Autodesk Inventor part; units mm, degrees
(part 2 of 4)
  line L908 (-4.5, 107.4545) -> (-3, 104.8564)
  line L909 (-7.5, 107.4545) -> (-4.5, 107.4545)
  line L910 (-9, 104.8564) -> (-7.5, 107.4545)
  line L911 (-11.5, 100.5263) -> (-8.5, 100.5263)
  line L912 (-3, 91) -> (-3, 104.8564) construction
  line L913 (-80.5, 109.3301) -> (-83.5, 109.3301)
  line L914 (-83.5, 109.3301) -> (-85, 111.9282)
  line L915 (-85, 111.9282) -> (-83.5, 114.5263)
  line L916 (-83.5, 114.5263) -> (-80.5, 114.5263)
  line L917 (-72.5, 109.3301) -> (-75.5, 109.3301)
  line L918 (-75.5, 109.3301) -> (-77, 111.9282)
  line L919 (-80.5, 114.5263) -> (-79, 111.9282)
  line L920 (-77, 111.9282) -> (-75.5, 114.5263)
  line L921 (-71, 111.9282) -> (-72.5, 109.3301)
  line L922 (-75.5, 114.5263) -> (-72.5, 114.5263)
  line L923 (-72.5, 114.5263) -> (-71, 111.9282)
  line L924 (-79, 111.9282) -> (-80.5, 109.3301)
  line L925 (-51.5, 114.5263) -> (-48.5, 114.5263)
  line L926 (-48.5, 109.3301) -> (-51.5, 109.3301)
  line L927 (-51.5, 109.3301) -> (-53, 111.9282)
  line L928 (-53, 111.9282) -> (-51.5, 114.5263)
  line L929 (-56.5, 114.5263) -> (-55, 111.9282)
  line L930 (-55, 111.9282) -> (-56.5, 109.3301)
  line L931 (-56.5, 109.3301) -> (-59.5, 109.3301)
  line L932 (-59.5, 114.5263) -> (-56.5, 114.5263)
  line L933 (-61, 111.9282) -> (-59.5, 114.5263)
  line L934 (-64.5, 114.5263) -> (-63, 111.9282)
  line L935 (-63, 111.9282) -> (-64.5, 109.3301)
  line L936 (-67.5, 114.5263) -> (-64.5, 114.5263)
  line L937 (-64.5, 109.3301) -> (-67.5, 109.3301)
  line L938 (-69, 111.9282) -> (-67.5, 114.5263)
  line L939 (-67.5, 109.3301) -> (-69, 111.9282)
  line L940 (-59.5, 109.3301) -> (-61, 111.9282)
  line L941 (-76.5, 116.2583) -> (-79.5, 116.2583)
  line L942 (-79.5, 116.2583) -> (-81, 118.8564)
  line L943 (-79.5, 121.4545) -> (-76.5, 121.4545)
  line L944 (-81, 118.8564) -> (-79.5, 121.4545)
  line L945 (-39.5, 116.2583) -> (-41, 118.8564)
  line L946 (-41, 118.8564) -> (-39.5, 121.4545)
  line L947 (-43, 118.8564) -> (-44.5, 116.2583)
  line L948 (-44.5, 121.4545) -> (-43, 118.8564)
  line L949 (-47.5, 121.4545) -> (-44.5, 121.4545)
  line L950 (-49, 118.8564) -> (-47.5, 121.4545)
  line L951 (-47.5, 116.2583) -> (-49, 118.8564)
  line L952 (-52.5, 121.4545) -> (-51, 118.8564)
  line L953 (-51, 118.8564) -> (-52.5, 116.2583)
  line L954 (-55.5, 121.4545) -> (-52.5, 121.4545)
  line L955 (-52.5, 116.2583) -> (-55.5, 116.2583)
  line L956 (-44.5, 116.2583) -> (-47.5, 116.2583)
  line L957 (-57, 118.8564) -> (-55.5, 121.4545)
  line L958 (-60.5, 121.4545) -> (-59, 118.8564)
  line L959 (-59, 118.8564) -> (-60.5, 116.2583)
  line L960 (-63.5, 121.4545) -> (-60.5, 121.4545)
  line L961 (-60.5, 116.2583) -> (-63.5, 116.2583)
  line L962 (-63.5, 116.2583) -> (-65, 118.8564)
  line L963 (-65, 118.8564) -> (-63.5, 121.4545)
  line L964 (-55.5, 116.2583) -> (-57, 118.8564)
  line L965 (-67, 118.8564) -> (-68.5, 116.2583)
  line L966 (-68.5, 121.4545) -> (-67, 118.8564)
  line L967 (-68.5, 116.2583) -> (-71.5, 116.2583)
  line L968 (-71.5, 116.2583) -> (-73, 118.8564)
  line L969 (-73, 118.8564) -> (-71.5, 121.4545)
  line L970 (-75, 118.8564) -> (-76.5, 116.2583)
  line L971 (-76.5, 121.4545) -> (-75, 118.8564)
  line L972 (-71.5, 121.4545) -> (-68.5, 121.4545)
  line L973 (-47, 111.9282) -> (-48.5, 109.3301)
  line L974 (-48.5, 114.5263) -> (-47, 111.9282)
  line L975 (-45, 111.9282) -> (-43.5, 114.5263)
  line L976 (-43.5, 109.3301) -> (-45, 111.9282)
  line L977 (-43.5, 114.5263) -> (-40.5, 114.5263)
  line L978 (-40.5, 109.3301) -> (-43.5, 109.3301)
  line L979 (-40.5, 114.5263) -> (-39, 111.9282)
  line L980 (-39, 111.9282) -> (-40.5, 109.3301)
  line L981 (-11, 118.8564) -> (-12.5, 116.2583)
  line L982 (-12.5, 121.4545) -> (-11, 118.8564)
  line L983 (-24.5, 114.5263) -> (-23, 111.9282)
  line L984 (-23, 111.9282) -> (-24.5, 109.3301)
  line L985 (-27.5, 114.5263) -> (-24.5, 114.5263)
  line L986 (-24.5, 109.3301) -> (-27.5, 109.3301)
  line L987 (-29, 111.9282) -> (-27.5, 114.5263)
  line L988 (-27.5, 109.3301) -> (-29, 111.9282)
  line L989 (-31, 111.9282) -> (-32.5, 109.3301)
  line L990 (-32.5, 114.5263) -> (-31, 111.9282)
  line L991 (-32.5, 109.3301) -> (-35.5, 109.3301)
  line L992 (-35.5, 114.5263) -> (-32.5, 114.5263)
  line L993 (-35.5, 109.3301) -> (-37, 111.9282)
  line L994 (-37, 111.9282) -> (-35.5, 114.5263)
  line L995 (-19.5, 109.3301) -> (-21, 111.9282)
  line L996 (-21, 111.9282) -> (-19.5, 114.5263)
  line L997 (-19.5, 114.5263) -> (-16.5, 114.5263)
  line L998 (-16.5, 109.3301) -> (-19.5, 109.3301)
  line L999 (-16.5, 114.5263) -> (-15, 111.9282)
  line L1000 (-15, 111.9282) -> (-16.5, 109.3301)
  line L1001 (-20.5, 116.2583) -> (-23.5, 116.2583)
  line L1002 (-23.5, 121.4545) -> (-20.5, 121.4545)
  line L1003 (-19, 118.8564) -> (-20.5, 116.2583)
  line L1004 (-20.5, 121.4545) -> (-19, 118.8564)
  line L1005 (-17, 118.8564) -> (-15.5, 121.4545)
  line L1006 (-15.5, 116.2583) -> (-17, 118.8564)
  line L1007 (-12.5, 116.2583) -> (-15.5, 116.2583)
  line L1008 (-15.5, 121.4545) -> (-12.5, 121.4545)
  line L1009 (-25, 118.8564) -> (-23.5, 121.4545)
  line L1010 (-28.5, 121.4545) -> (-27, 118.8564)
  line L1011 (-27, 118.8564) -> (-28.5, 116.2583)
  line L1012 (-31.5, 121.4545) -> (-28.5, 121.4545)
  line L1013 (-28.5, 116.2583) -> (-31.5, 116.2583)
  line L1014 (-33, 118.8564) -> (-31.5, 121.4545)
  line L1015 (-31.5, 116.2583) -> (-33, 118.8564)
  line L1016 (-23.5, 116.2583) -> (-25, 118.8564)
  line L1017 (-36.5, 121.4545) -> (-35, 118.8564)
  line L1018 (-35, 118.8564) -> (-36.5, 116.2583)
  line L1019 (-39.5, 121.4545) -> (-36.5, 121.4545)
  line L1020 (-36.5, 116.2583) -> (-39.5, 116.2583)
  line L1021 (-13, 111.9282) -> (-11.5, 114.5263)
  line L1022 (-8.5, 109.3301) -> (-11.5, 109.3301)
  line L1023 (-11.5, 109.3301) -> (-13, 111.9282)
  line L1024 (-8.5, 114.5263) -> (-7, 111.9282)
  line L1025 (-7, 111.9282) -> (-8.5, 109.3301)
  line L1026 (-4.5, 116.2583) -> (-7.5, 116.2583)
  line L1027 (-7.5, 116.2583) -> (-9, 118.8564)
  line L1028 (-3, 118.8564) -> (-4.5, 116.2583)
  line L1029 (-4.5, 121.4545) -> (-3, 118.8564)
  line L1030 (-7.5, 121.4545) -> (-4.5, 121.4545)
  line L1031 (-9, 118.8564) -> (-7.5, 121.4545)
  line L1032 (-11.5, 114.5263) -> (-8.5, 114.5263)
  line L1033 (-3, 105) -> (-3, 118.8564) construction
  line L1034 (-80.5, 123.3301) -> (-83.5, 123.3301)
  line L1035 (-83.5, 123.3301) -> (-85, 125.9282)
  line L1036 (-85, 125.9282) -> (-83.5, 128.5263)
  line L1037 (-83.5, 128.5263) -> (-80.5, 128.5263)
  line L1038 (-72.5, 123.3301) -> (-75.5, 123.3301)
  line L1039 (-75.5, 123.3301) -> (-77, 125.9282)
  line L1040 (-80.5, 128.5263) -> (-79, 125.9282)
  line L1041 (-77, 125.9282) -> (-75.5, 128.5263)
  line L1042 (-71, 125.9282) -> (-72.5, 123.3301)
  line L1043 (-75.5, 128.5263) -> (-72.5, 128.5263)
  line L1044 (-72.5, 128.5263) -> (-71, 125.9282)
  line L1045 (-79, 125.9282) -> (-80.5, 123.3301)
  line L1046 (-51.5, 128.5263) -> (-48.5, 128.5263)
  line L1047 (-48.5, 123.3301) -> (-51.5, 123.3301)
  line L1048 (-51.5, 123.3301) -> (-53, 125.9282)
  line L1049 (-53, 125.9282) -> (-51.5, 128.5263)
  line L1050 (-56.5, 128.5263) -> (-55, 125.9282)
  line L1051 (-55, 125.9282) -> (-56.5, 123.3301)
  line L1052 (-56.5, 123.3301) -> (-59.5, 123.3301)
  line L1053 (-59.5, 128.5263) -> (-56.5, 128.5263)
  line L1054 (-61, 125.9282) -> (-59.5, 128.5263)
  line L1055 (-64.5, 128.5263) -> (-63, 125.9282)
  line L1056 (-63, 125.9282) -> (-64.5, 123.3301)
  line L1057 (-67.5, 128.5263) -> (-64.5, 128.5263)
  line L1058 (-64.5, 123.3301) -> (-67.5, 123.3301)
  line L1059 (-69, 125.9282) -> (-67.5, 128.5263)
  line L1060 (-67.5, 123.3301) -> (-69, 125.9282)
  line L1061 (-59.5, 123.3301) -> (-61, 125.9282)
  line L1062 (-76.5, 130.2583) -> (-79.5, 130.2583)
  line L1063 (-79.5, 130.2583) -> (-81, 132.8564)
  line L1064 (-79.5, 135.4545) -> (-76.5, 135.4545)
  line L1065 (-81, 132.8564) -> (-79.5, 135.4545)
  line L1066 (-39.5, 130.2583) -> (-41, 132.8564)
  line L1067 (-41, 132.8564) -> (-39.5, 135.4545)
  line L1068 (-43, 132.8564) -> (-44.5, 130.2583)
  line L1069 (-44.5, 135.4545) -> (-43, 132.8564)
  line L1070 (-47.5, 135.4545) -> (-44.5, 135.4545)
  line L1071 (-49, 132.8564) -> (-47.5, 135.4545)
  line L1072 (-47.5, 130.2583) -> (-49, 132.8564)
  line L1073 (-52.5, 135.4545) -> (-51, 132.8564)
  line L1074 (-51, 132.8564) -> (-52.5, 130.2583)
  line L1075 (-55.5, 135.4545) -> (-52.5, 135.4545)
  line L1076 (-52.5, 130.2583) -> (-55.5, 130.2583)
  line L1077 (-44.5, 130.2583) -> (-47.5, 130.2583)
  line L1078 (-57, 132.8564) -> (-55.5, 135.4545)
  line L1079 (-60.5, 135.4545) -> (-59, 132.8564)
  line L1080 (-59, 132.8564) -> (-60.5, 130.2583)
  line L1081 (-63.5, 135.4545) -> (-60.5, 135.4545)
  line L1082 (-60.5, 130.2583) -> (-63.5, 130.2583)
  line L1083 (-63.5, 130.2583) -> (-65, 132.8564)
  line L1084 (-65, 132.8564) -> (-63.5, 135.4545)
  line L1085 (-55.5, 130.2583) -> (-57, 132.8564)
  line L1086 (-67, 132.8564) -> (-68.5, 130.2583)
  line L1087 (-68.5, 135.4545) -> (-67, 132.8564)
  line L1088 (-68.5, 130.2583) -> (-71.5, 130.2583)
  line L1089 (-71.5, 130.2583) -> (-73, 132.8564)
  line L1090 (-73, 132.8564) -> (-71.5, 135.4545)
  line L1091 (-75, 132.8564) -> (-76.5, 130.2583)
  line L1092 (-76.5, 135.4545) -> (-75, 132.8564)
  line L1093 (-71.5, 135.4545) -> (-68.5, 135.4545)
  line L1094 (-47, 125.9282) -> (-48.5, 123.3301)
  line L1095 (-48.5, 128.5263) -> (-47, 125.9282)
  line L1096 (-45, 125.9282) -> (-43.5, 128.5263)
  line L1097 (-43.5, 123.3301) -> (-45, 125.9282)
  line L1098 (-43.5, 128.5263) -> (-40.5, 128.5263)
  line L1099 (-40.5, 123.3301) -> (-43.5, 123.3301)
  line L1100 (-40.5, 128.5263) -> (-39, 125.9282)
  line L1101 (-39, 125.9282) -> (-40.5, 123.3301)
  line L1102 (-11, 132.8564) -> (-12.5, 130.2583)
  line L1103 (-12.5, 135.4545) -> (-11, 132.8564)
  line L1104 (-24.5, 128.5263) -> (-23, 125.9282)
  line L1105 (-23, 125.9282) -> (-24.5, 123.3301)
  line L1106 (-27.5, 128.5263) -> (-24.5, 128.5263)
  line L1107 (-24.5, 123.3301) -> (-27.5, 123.3301)
  line L1108 (-29, 125.9282) -> (-27.5, 128.5263)
  line L1109 (-27.5, 123.3301) -> (-29, 125.9282)
  line L1110 (-31, 125.9282) -> (-32.5, 123.3301)
  line L1111 (-32.5, 128.5263) -> (-31, 125.9282)
  line L1112 (-32.5, 123.3301) -> (-35.5, 123.3301)
  line L1113 (-35.5, 128.5263) -> (-32.5, 128.5263)
  line L1114 (-35.5, 123.3301) -> (-37, 125.9282)
  line L1115 (-37, 125.9282) -> (-35.5, 128.5263)
  line L1116 (-19.5, 123.3301) -> (-21, 125.9282)
  line L1117 (-21, 125.9282) -> (-19.5, 128.5263)
  line L1118 (-19.5, 128.5263) -> (-16.5, 128.5263)
  line L1119 (-16.5, 123.3301) -> (-19.5, 123.3301)
  line L1120 (-16.5, 128.5263) -> (-15, 125.9282)
  line L1121 (-15, 125.9282) -> (-16.5, 123.3301)
  line L1122 (-20.5, 130.2583) -> (-23.5, 130.2583)
  line L1123 (-23.5, 135.4545) -> (-20.5, 135.4545)
  line L1124 (-19, 132.8564) -> (-20.5, 130.2583)
  line L1125 (-20.5, 135.4545) -> (-19, 132.8564)
  line L1126 (-17, 132.8564) -> (-15.5, 135.4545)
  line L1127 (-15.5, 130.2583) -> (-17, 132.8564)
  line L1128 (-12.5, 130.2583) -> (-15.5, 130.2583)
  line L1129 (-15.5, 135.4545) -> (-12.5, 135.4545)
  line L1130 (-25, 132.8564) -> (-23.5, 135.4545)
  line L1131 (-28.5, 135.4545) -> (-27, 132.8564)
  line L1132 (-27, 132.8564) -> (-28.5, 130.2583)
  line L1133 (-31.5, 135.4545) -> (-28.5, 135.4545)
  line L1134 (-28.5, 130.2583) -> (-31.5, 130.2583)
  line L1135 (-33, 132.8564) -> (-31.5, 135.4545)
  line L1136 (-31.5, 130.2583) -> (-33, 132.8564)
  line L1137 (-23.5, 130.2583) -> (-25, 132.8564)
  line L1138 (-36.5, 135.4545) -> (-35, 132.8564)
  line L1139 (-35, 132.8564) -> (-36.5, 130.2583)
  line L1140 (-39.5, 135.4545) -> (-36.5, 135.4545)
  line L1141 (-36.5, 130.2583) -> (-39.5, 130.2583)
  line L1142 (-13, 125.9282) -> (-11.5, 128.5263)
  line L1143 (-8.5, 123.3301) -> (-11.5, 123.3301)
  line L1144 (-11.5, 123.3301) -> (-13, 125.9282)
  line L1145 (-8.5, 128.5263) -> (-7, 125.9282)
  line L1146 (-7, 125.9282) -> (-8.5, 123.3301)
  line L1147 (-4.5, 130.2583) -> (-7.5, 130.2583)
  line L1148 (-7.5, 130.2583) -> (-9, 132.8564)
  line L1149 (-3, 132.8564) -> (-4.5, 130.2583)
  line L1150 (-4.5, 135.4545) -> (-3, 132.8564)
  line L1151 (-7.5, 135.4545) -> (-4.5, 135.4545)
  line L1152 (-9, 132.8564) -> (-7.5, 135.4545)
  line L1153 (-11.5, 128.5263) -> (-8.5, 128.5263)
  line L1154 (-3, 119) -> (-3, 132.8564) construction
  point P0 (0, 75)
  point P1 (-6, 7)
  point P2 (-14, 7)
  point P3 (-22, 7)
  point P4 (-30, 7)
  point P5 (-38, 7)
  point P6 (-46, 7)
  point P7 (-54, 7)
  point P8 (-62, 7)
  point P9 (-70, 7)
  point P10 (-78, 7)
  point P11 (-10, 13.9282)
  point P12 (-18, 13.9282)
  point P13 (-26, 13.9282)
  point P14 (-34, 13.9282)
  point P15 (-42, 13.9282)
  point P16 (-50, 13.9282)
  point P17 (-58, 13.9282)
  point P18 (-66, 13.9282)
  point P19 (-74, 13.9282)
  point P20 (-82, 13.9282)
  point P21 (-14, 20.8564)
  point P22 (-22, 20.8564)
  point P23 (-30, 20.8564)
  point P24 (-38, 20.8564)
  point P25 (-46, 20.8564)
  point P26 (-54, 20.8564)
  point P27 (-62, 20.8564)
  point P28 (-70, 20.8564)
  point P29 (-78, 20.8564)
  point P30 (-86, 20.8564)
  point P31 (-6, 20.8564)
  point P32 (-82, 27.9282)
  point P33 (-74, 27.9282)
  point P34 (-50, 27.9282)
  point P35 (-58, 27.9282)
  point P36 (-66, 27.9282)
  point P37 (-84.5, 32.2583)
  point P38 (-83, 34.8564)
  point P39 (-86, 34.8564)
  point P40 (-84.5, 37.4545)
  point P41 (-78, 34.8564)
  point P42 (-46, 34.8564)
  point P43 (-54, 34.8564)
  point P44 (-62, 34.8564)
  point P45 (-70, 34.8564)
  point P46 (-42, 27.9282)
  point P47 (-26, 27.9282)
  point P48 (-34, 27.9282)
  point P49 (-18, 27.9282)
  point P50 (-14, 34.8564)
  point P51 (-22, 34.8564)
  point P52 (-30, 34.8564)
  point P53 (-38, 34.8564)
  point P54 (-10, 27.9282)
  point P55 (-6, 34.8564)
  point P56 (-82, 41.9282)
  point P57 (-74, 41.9282)
  point P58 (-50, 41.9282)
  point P59 (-58, 41.9282)
  point P60 (-66, 41.9282)
  point P61 (-84.5, 46.2583)
  point P62 (-83, 48.8564)
  point P63 (-86, 48.8564)
  point P64 (-84.5, 51.4545)
  point P65 (-78, 48.8564)
  point P66 (-46, 48.8564)
  point P67 (-54, 48.8564)
  point P68 (-62, 48.8564)
  point P69 (-70, 48.8564)
  point P70 (-42, 41.9282)
  point P71 (-26, 41.9282)
  point P72 (-34, 41.9282)
  point P73 (-18, 41.9282)
  point P74 (-14, 48.8564)
  point P75 (-22, 48.8564)
  point P76 (-30, 48.8564)
  point P77 (-38, 48.8564)
  point P78 (-10, 41.9282)
  point P79 (-6, 48.8564)
  point P80 (-82, 55.9282)
  point P81 (-74, 55.9282)
  point P82 (-50, 55.9282)
  point P83 (-58, 55.9282)
  point P84 (-66, 55.9282)
  point P85 (-84.5, 60.2583)
  point P86 (-83, 62.8564)
  point P87 (-86, 62.8564)
  point P88 (-84.5, 65.4545)
  point P89 (-78, 62.8564)
  point P90 (-46, 62.8564)
  point P91 (-54, 62.8564)
  point P92 (-62, 62.8564)
  point P93 (-70, 62.8564)
  point P94 (-42, 55.9282)
  point P95 (-26, 55.9282)
  point P96 (-34, 55.9282)
  point P97 (-18, 55.9282)
  point P98 (-14, 62.8564)
  point P99 (-22, 62.8564)
  point P100 (-30, 62.8564)
  point P101 (-38, 62.8564)
  point P102 (-10, 55.9282)
  point P103 (-6, 62.8564)
  point P104 (-82, 69.9282)
  point P105 (-74, 69.9282)
  point P106 (-50, 69.9282)
  point P107 (-58, 69.9282)
  point P108 (-66, 69.9282)
  point P109 (-84.5, 74.2583)
  point P110 (-83, 76.8564)
  point P111 (-86, 76.8564)
  point P112 (-84.5, 79.4545)
  point P113 (-78, 76.8564)
  point P114 (-46, 76.8564)
  point P115 (-54, 76.8564)
  point P116 (-62, 76.8564)
  point P117 (-70, 76.8564)
  point P118 (-42, 69.9282)
  point P119 (-26, 69.9282)
  point P120 (-34, 69.9282)
  point P121 (-18, 69.9282)
  point P122 (-14, 76.8564)
  point P123 (-22, 76.8564)
  point P124 (-30, 76.8564)
  point P125 (-38, 76.8564)
  point P126 (-10, 69.9282)
  point P127 (-6, 76.8564)
  point P128 (-82, 83.9282)
  point P129 (-74, 83.9282)
  point P130 (-50, 83.9282)
  point P131 (-58, 83.9282)
  point P132 (-66, 83.9282)
  point P133 (-84.5, 88.2583)
  point P134 (-83, 90.8564)
  point P135 (-86, 90.8564)
  point P136 (-84.5, 93.4545)
  point P137 (-78, 90.8564)
  point P138 (-46, 90.8564)
  point P139 (-54, 90.8564)
  point P140 (-62, 90.8564)
  point P141 (-70, 90.8564)
  point P142 (-42, 83.9282)
  point P143 (-26, 83.9282)
  point P144 (-34, 83.9282)
  point P145 (-18, 83.9282)
  point P146 (-14, 90.8564)
  point P147 (-22, 90.8564)
  point P148 (-30, 90.8564)
  point P149 (-38, 90.8564)
  point P150 (-10, 83.9282)
  point P151 (-6, 90.8564)
  point P152 (-82, 97.9282)
  point P153 (-74, 97.9282)
  point P154 (-50, 97.9282)
  point P155 (-58, 97.9282)
  point P156 (-66, 97.9282)
  point P157 (-84.5, 102.2583)
  point P158 (-83, 104.8564)
  point P159 (-86, 104.8564)
  point P160 (-84.5, 107.4545)
  point P161 (-78, 104.8564)
  point P162 (-46, 104.8564)
  point P163 (-54, 104.8564)
  point P164 (-62, 104.8564)
  point P165 (-70, 104.8564)
  point P166 (-42, 97.9282)
  point P167 (-26, 97.9282)
  point P168 (-34, 97.9282)
  point P169 (-18, 97.9282)
  point P170 (-14, 104.8564)
  point P171 (-22, 104.8564)
  point P172 (-30, 104.8564)
  point P173 (-38, 104.8564)
  point P174 (-10, 97.9282)
  point P175 (-6, 104.8564)
  point P176 (-82, 111.9282)
  point P177 (-74, 111.9282)
  point P178 (-50, 111.9282)
  point P179 (-58, 111.9282)
  point P180 (-66, 111.9282)
  point P181 (-84.5, 116.2583)
  point P182 (-83, 118.8564)
  point P183 (-86, 118.8564)
  point P184 (-84.5, 121.4545)
  point P185 (-78, 118.8564)
  point P186 (-46, 118.8564)
  point P187 (-54, 118.8564)
  point P188 (-62, 118.8564)
  point P189 (-70, 118.8564)
  point P190 (-42, 111.9282)
  point P191 (-26, 111.9282)
  point P192 (-34, 111.9282)
  point P193 (-18, 111.9282)
  point P194 (-14, 118.8564)
  point P195 (-22, 118.8564)
  point P196 (-30, 118.8564)
  point P197 (-38, 118.8564)
  point P198 (-10, 111.9282)
  point P199 (-6, 118.8564)
  dimension "d22" = 3
  dimension "d25" = 8
  dimension "d28" = 8
  dimension "d33" = 8
  dimension "d40" = 14
  constraints: 2310 end point, 4 collinear, 2 horizontal, 2 vertical, 2528 other
  measures "d22" distance of point (-6, 7) L0.start
  measures "d25" distance of point (-6, 7) point (-14, 7)
  measures "d28" distance of point (-6, 7) point (-10, 13.928)
  measures "d33" distance of point (-14, 20.856) point (-6, 20.856)
  measures "d40" distance of L117.end L187.start
extrude "Estrusione3" cut sketch "Schizzo4" against normal blind 5 contours L12 L13 L14 L15 L16 L17 | L18 L19 L20 L21 L22 L23 | L24 L25 L26 L27 L28 L29 | L30 L31 L32 L33 L34 L35 | L36 L37 L38 L39 L40 L41 | L42 L43 L44 L45 L46 L47 | L48 L49 L50 L51 L52 L53 | L60 L61 L62 L63 L64 L65 | L66 L67 L68 L69 L70 L71 | L72 L73 L74 L75 L76 L77 | L78 L79 L80 L81 L82 L83 | L84 L85 L86 L87 L88 L89 | L90 L91 L92 L93 L94 L95 | L96 L97 L98 L99 L100 L101 | L102 L103 L104 L105 L106 L107 | L108 L109 L110 L111 L112 L113 | L114 L115 L116 L117 L118 L119 | L120 L121 L122 L123 L124 L125 | L126 L127 L128 L129 L130 L131 | L132 L133 L134 L135 L136 L137 | L138 L139 L140 L141 L142 L143 | L144 L145 L146 L147 L148 L149 | L150 L151 L152 L153 L154 L155 | L156 L157 L158 L159 L160 L161 | L162 L163 L164 L165 L166 L167 | L168 L169 L170 L171 L172 L173 | L180 L182 L185 L184 L183 L181 | L187 L188 L189 L190 L193 L198 | L191 L192 L194 L196 L197 L195 | L199 L248 L247 L200 L201 L202 | L203 L204 L205 L214 L207 L206 | L208 L209 L211 L213 L212 L210 | L215 L216 L218 L217 L245 L244 | L219 L220 L293 L291 L292 L294 | L221 L230 L225 L224 L223 L222 | L226 L227 L229 L238 L231 L228 | L232 L233 L235 L236 L237 L234 | L239 L241 L242 L243 L246 L240 | L249 L251 L253 L254 L252 L250 | L255 L281 L280 L279 L282 L256 | L257 L258 L260 L262 L261 L259 | L263 L265 L267 L268 L266 L264 | L269 L270 L271 L273 L274 L272 | L275 L290 L283 L276 L278 L277 | L284 L285 L287 L289 L288 L286 | L295 L306 L298 L299 L296 L297 | L300 L301 L305 L304 L303 L302 | L308 L309 L310 L311 L314 L319 | L312 L313 L315 L317 L318 L316 | L320 L369 L368 L321 L322 L323 | L324 L325 L326 L335 L328 L327 | L329 L330 L332 L334 L333 L331 | L336 L337 L339 L338 L366 L365 | L340 L341 L414 L412 L413 L415 | L342 L351 L346 L345 L344 L343 | L347 L348 L350 L359 L352 L349 | L353 L354 L356 L357 L358 L355 | L360 L362 L363 L364 L367 L361 | L370 L372 L374 L375 L373 L371 | L376 L402 L401 L400 L403 L377 | L378 L379 L381 L383 L382 L380 | L384 L386 L388 L389 L387 L385 | L390 L391 L392 L394 L395 L393 | L396 L411 L404 L397 L399 L398 | L405 L406 L408 L410 L409 L407 | L416 L427 L419 L420 L417 L418 | L421 L422 L426 L425 L424 L423 | L429 L430 L431 L432 L435 L440 | L433 L434 L436 L438 L439 L437 | L441 L490 L489 L442 L443 L444 | L445 L446 L447 L456 L449 L448 | L450 L451 L453 L455 L454 L452 | L457 L458 L460 L459 L487 L486 | L461 L462 L535 L533 L534 L536 | L463 L472 L467 L466 L465 L464 | L468 L469 L471 L480 L473 L470 | L474 L475 L477 L478 L479 L476 | L481 L483 L484 L485 L488 L482 | L491 L493 L495 L496 L494 L492 | L497 L523 L522 L521 L524 L498 | L499 L500 L502 L504 L503 L501 | L505 L507 L509 L510 L508 L506 | L511 L512 L513 L515 L516 L514 | L517 L532 L525 L518 L520 L519 | L526 L527 L529 L531 L530 L528 | L537 L548 L540 L541 L538 L539 | L542 L543 L547 L546 L545 L544 | L550 L551 L552 L553 L556 L561 | L554 L555 L557 L559 L560 L558 | L562 L611 L610 L563 L564 L565 | L566 L567 L568 L577 L570 L569 | L571 L572 L574 L576 L575 L573 | L578 L579 L581 L580 L608 L607 | L582 L583 L656 L654 L655 L657 | L584 L593 L588 L587 L586 L585 | L589 L590 L592 L601 L594 L591 | L595 L596 L598 L599 L600 L597 | L602 L604 L605 L606 L609 L603 | L612 L614 L616 L617 L615 L613 | L618 L644 L643 L642 L645 L619 | L620 L621 L623 L625 L624 L622 | L626 L628 L630 L631 L629 L627 | L632 L633 L634 L636 L637 L635 | L638 L653 L646 L639 L641 L640 | L647 L648 L650 L652 L651 L649 | L658 L669 L661 L662 L659 L660 | L663 L664 L668 L667 L666 L665 | L671 L672 L673 L674 L677 L682 | L675 L676 L678 L680 L681 L679 | L683 L732 L731 L684 L685 L686 | L687 L688 L689 L698 L691 L690 | L692 L693 L695 L697 L696 L694 | L699 L700 L702 L701 L729 L728 | L703 L704 L777 L775 L776 L778 | L705 L714 L709 L708 L707 L706 | L710 L711 L713 L722 L715 L712 | L716 L717 L719 L720 L721 L718 | L723 L725 L726 L727 L730 L724 | L733 L735 L737 L738 L736 L734 | L741 L742 L744 L746 L745 L743 | L747 L749 L751 L752 L750 L748 | L753 L754 L755 L757 L758 L756 | L779 L790 L782 L783 L780 L781 | L792 L793 L794 L795 L798 L803 | L796 L797 L799 L801 L802 L800 | L804 L853 L852 L805 L806 L807 | L808 L809 L810 L819 L812 L811 | L813 L814 L816 L818 L817 L815 | L820 L821 L823 L822 L850 L849 | L824 L825 L898 L896 L897 L899 | L826 L835 L830 L829 L828 L827 | L831 L832 L834 L843 L836 L833 | L837 L838 L840 L841 L842 L839 | L844 L846 L847 L848 L851 L845 | L854 L856 L858 L859 L857 L855 | L868 L870 L872 L873 L871 L869 | L913 L914 L915 L916 L919 L924 | L917 L918 L920 L922 L923 L921 | L925 L974 L973 L926 L927 L928 | L929 L930 L931 L940 L933 L932 | L934 L935 L937 L939 L938 L936 | L941 L942 L944 L943 L971 L970 | L945 L946 L1019 L1017 L1018 L1020 | L947 L956 L951 L950 L949 L948 | L952 L953 L955 L964 L957 L954 | L958 L959 L961 L962 L963 L960 | L965 L967 L968 L969 L972 L966 | L975 L977 L979 L980 L978 L976 | L989 L991 L993 L994 L992 L990 | L1034 L1035 L1036 L1037 L1040 L1045 | L1038 L1039 L1041 L1043 L1044 L1042 | L1046 L1095 L1094 L1047 L1048 L1049 | L1050 L1051 L1052 L1061 L1054 L1053 | L1055 L1056 L1058 L1060 L1059 L1057 | L1066 L1067 L1140 L1138 L1139 L1141 | L1068 L1077 L1072 L1071 L1070 L1069 | L1073 L1074 L1076 L1085 L1078 L1075 | L1079 L1080 L1082 L1083 L1084 L1081 | L1086 L1088 L1089 L1090 L1093 L1087 | L1096 L1098 L1100 L1101 L1099 L1097 | L1110 L1112 L1114 L1115 L1113 L1111
sketch "Schizzo5" plane through (-70, -75, 0) normal (0, -1, 0) x (1, 0, 0)
  line L0 (140, 0) -> (0, 0)
  line L1 (140, 0) -> (140, 86)
  line L2 (0, 86) -> (140, 86)
  line L3 (0, 0) -> (0, 86)
  line L4 (125, 71) -> (125, 15)
  line L5 (125, 15) -> (15, 15)
  line L6 (15, 15) -> (15, 71)
  line L7 (15, 71) -> (125, 71)
  point P0 (70, 0)
  constraints: 8 end point, 3 other
extrude "Estrusione4" cut sketch "Schizzo5" against normal blind 1 contours L4 L5 L6 L7
sketch "Schizzo6" plane through (70, -75, 0) normal (1, 0, 0) x (0, 0, -1)
  line L0 (-39, 125.9282) -> (-40.5, 128.5263)
  line L1 (-40.5, 128.5263) -> (-43.5, 128.5263)
  line L2 (-43.5, 128.5263) -> (-45, 125.9282)
  line L3 (-45, 125.9282) -> (-43.5, 123.3301)
  line L4 (-43.5, 123.3301) -> (-40.5, 123.3301)
  line L5 (-40.5, 123.3301) -> (-39, 125.9282)
  line L6 (-63.5, 130.2583) -> (-60.5, 130.2583)
  line L7 (-60.5, 130.2583) -> (-59, 132.8564)
  line L8 (-59, 132.8564) -> (-60.5, 135.4545)
  line L9 (-60.5, 135.4545) -> (-63.5, 135.4545)
  line L10 (-63.5, 135.4545) -> (-65, 132.8564)
  line L11 (-65, 132.8564) -> (-63.5, 130.2583)
  line L12 (-47.5, 130.2583) -> (-44.5, 130.2583)
  line L13 (-44.5, 130.2583) -> (-43, 132.8564)
  line L14 (-43, 132.8564) -> (-44.5, 135.4545)
  line L15 (-44.5, 135.4545) -> (-47.5, 135.4545)
  line L16 (-47.5, 135.4545) -> (-49, 132.8564)
  line L17 (-49, 132.8564) -> (-47.5, 130.2583)
  line L18 (-59.5, 123.3301) -> (-56.5, 123.3301)
  line L19 (-56.5, 123.3301) -> (-55, 125.9282)
  line L20 (-55, 125.9282) -> (-56.5, 128.5263)
  line L21 (-56.5, 128.5263) -> (-59.5, 128.5263)
  line L22 (-59.5, 128.5263) -> (-61, 125.9282)
  line L23 (-61, 125.9282) -> (-59.5, 123.3301)
  line L24 (-71, 125.9282) -> (-72.5, 128.5263)
  line L25 (-72.5, 128.5263) -> (-75.5, 128.5263)
  line L26 (-75.5, 128.5263) -> (-77, 125.9282)
  line L27 (-77, 125.9282) -> (-75.5, 123.3301)
  line L28 (-75.5, 123.3301) -> (-72.5, 123.3301)
  line L29 (-72.5, 123.3301) -> (-71, 125.9282)
  line L30 (-35.5, 109.3301) -> (-32.5, 109.3301)
  line L31 (-32.5, 109.3301) -> (-31, 111.9282)
  line L32 (-31, 111.9282) -> (-32.5, 114.5263)
  line L33 (-32.5, 114.5263) -> (-35.5, 114.5263)
  line L34 (-35.5, 114.5263) -> (-37, 111.9282)
  line L35 (-37, 111.9282) -> (-35.5, 109.3301)
  line L36 (-71.5, 116.2583) -> (-68.5, 116.2583)
  line L37 (-68.5, 116.2583) -> (-67, 118.8564)
  line L38 (-67, 118.8564) -> (-68.5, 121.4545)
  line L39 (-68.5, 121.4545) -> (-71.5, 121.4545)
  line L40 (-71.5, 121.4545) -> (-73, 118.8564)
  line L41 (-73, 118.8564) -> (-71.5, 116.2583)
  line L42 (-55.5, 116.2583) -> (-52.5, 116.2583)
  line L43 (-52.5, 116.2583) -> (-51, 118.8564)
  line L44 (-51, 118.8564) -> (-52.5, 121.4545)
  line L45 (-52.5, 121.4545) -> (-55.5, 121.4545)
  line L46 (-55.5, 121.4545) -> (-57, 118.8564)
  line L47 (-57, 118.8564) -> (-55.5, 116.2583)
  line L48 (-39.5, 121.4545) -> (-41, 118.8564)
  line L49 (-41, 118.8564) -> (-39.5, 116.2583)
  line L50 (-39.5, 116.2583) -> (-36.5, 116.2583)
  line L51 (-36.5, 116.2583) -> (-35, 118.8564)
  line L52 (-35, 118.8564) -> (-36.5, 121.4545)
  line L53 (-36.5, 121.4545) -> (-39.5, 121.4545)
  line L54 (-67.5, 109.3301) -> (-64.5, 109.3301)
  line L55 (-64.5, 109.3301) -> (-63, 111.9282)
  line L56 (-63, 111.9282) -> (-64.5, 114.5263)
  line L57 (-64.5, 114.5263) -> (-67.5, 114.5263)
  line L58 (-67.5, 114.5263) -> (-69, 111.9282)
  line L59 (-69, 111.9282) -> (-67.5, 109.3301)
  line L60 (-47, 111.9282) -> (-48.5, 114.5263)
  line L61 (-48.5, 114.5263) -> (-51.5, 114.5263)
  line L62 (-51.5, 114.5263) -> (-53, 111.9282)
  line L63 (-53, 111.9282) -> (-51.5, 109.3301)
  line L64 (-51.5, 109.3301) -> (-48.5, 109.3301)
  line L65 (-48.5, 109.3301) -> (-47, 111.9282)
  line L66 (-80.5, 114.5263) -> (-83.5, 114.5263)
  line L67 (-83.5, 114.5263) -> (-85, 111.9282)
  line L68 (-85, 111.9282) -> (-83.5, 109.3301)
  line L69 (-83.5, 109.3301) -> (-80.5, 109.3301)
  line L70 (-80.5, 109.3301) -> (-79, 111.9282)
  line L71 (-79, 111.9282) -> (-80.5, 114.5263)
  line L72 (-39, 97.9282) -> (-40.5, 100.5263)
  line L73 (-40.5, 100.5263) -> (-43.5, 100.5263)
  line L74 (-43.5, 100.5263) -> (-45, 97.9282)
  line L75 (-45, 97.9282) -> (-43.5, 95.3301)
  line L76 (-43.5, 95.3301) -> (-40.5, 95.3301)
  line L77 (-40.5, 95.3301) -> (-39, 97.9282)
  line L78 (-63.5, 102.2583) -> (-60.5, 102.2583)
  line L79 (-60.5, 102.2583) -> (-59, 104.8564)
  line L80 (-59, 104.8564) -> (-60.5, 107.4545)
  line L81 (-60.5, 107.4545) -> (-63.5, 107.4545)
  line L82 (-63.5, 107.4545) -> (-65, 104.8564)
  line L83 (-65, 104.8564) -> (-63.5, 102.2583)
  line L84 (-47.5, 102.2583) -> (-44.5, 102.2583)
  line L85 (-44.5, 102.2583) -> (-43, 104.8564)
  line L86 (-43, 104.8564) -> (-44.5, 107.4545)
  line L87 (-44.5, 107.4545) -> (-47.5, 107.4545)
  line L88 (-47.5, 107.4545) -> (-49, 104.8564)
  line L89 (-49, 104.8564) -> (-47.5, 102.2583)
  line L90 (-79.5, 107.4545) -> (-81, 104.8564)
  line L91 (-81, 104.8564) -> (-79.5, 102.2583)
  line L92 (-79.5, 102.2583) -> (-76.5, 102.2583)
  line L93 (-76.5, 102.2583) -> (-75, 104.8564)
  line L94 (-75, 104.8564) -> (-76.5, 107.4545)
  line L95 (-76.5, 107.4545) -> (-79.5, 107.4545)
  line L96 (-59.5, 95.3301) -> (-56.5, 95.3301)
  line L97 (-56.5, 95.3301) -> (-55, 97.9282)
  line L98 (-55, 97.9282) -> (-56.5, 100.5263)
  line L99 (-56.5, 100.5263) -> (-59.5, 100.5263)
  line L100 (-59.5, 100.5263) -> (-61, 97.9282)
  line L101 (-61, 97.9282) -> (-59.5, 95.3301)
  line L102 (-71, 97.9282) -> (-72.5, 100.5263)
  line L103 (-72.5, 100.5263) -> (-75.5, 100.5263)
  line L104 (-75.5, 100.5263) -> (-77, 97.9282)
  line L105 (-77, 97.9282) -> (-75.5, 95.3301)
  line L106 (-75.5, 95.3301) -> (-72.5, 95.3301)
  line L107 (-72.5, 95.3301) -> (-71, 97.9282)
  line L108 (-7, 83.9282) -> (-8.5, 86.5263)
  line L109 (-8.5, 86.5263) -> (-11.5, 86.5263)
  line L110 (-11.5, 86.5263) -> (-13, 83.9282)
  line L111 (-13, 83.9282) -> (-11.5, 81.3301)
  line L112 (-11.5, 81.3301) -> (-8.5, 81.3301)
  line L113 (-8.5, 81.3301) -> (-7, 83.9282)
  line L114 (-35.5, 81.3301) -> (-32.5, 81.3301)
  line L115 (-32.5, 81.3301) -> (-31, 83.9282)
  line L116 (-31, 83.9282) -> (-32.5, 86.5263)
  line L117 (-32.5, 86.5263) -> (-35.5, 86.5263)
  line L118 (-35.5, 86.5263) -> (-37, 83.9282)
  line L119 (-37, 83.9282) -> (-35.5, 81.3301)
  line L120 (-39, 83.9282) -> (-40.5, 86.5263)
  line L121 (-40.5, 86.5263) -> (-43.5, 86.5263)
  line L122 (-43.5, 86.5263) -> (-45, 83.9282)
  line L123 (-45, 83.9282) -> (-43.5, 81.3301)
  line L124 (-43.5, 81.3301) -> (-40.5, 81.3301)
  line L125 (-40.5, 81.3301) -> (-39, 83.9282)
  line L126 (-63.5, 88.2583) -> (-60.5, 88.2583)
  line L127 (-60.5, 88.2583) -> (-59, 90.8564)
  line L128 (-59, 90.8564) -> (-60.5, 93.4545)
  line L129 (-60.5, 93.4545) -> (-63.5, 93.4545)
  line L130 (-63.5, 93.4545) -> (-65, 90.8564)
  line L131 (-65, 90.8564) -> (-63.5, 88.2583)
  line L132 (-47.5, 88.2583) -> (-44.5, 88.2583)
  line L133 (-44.5, 88.2583) -> (-43, 90.8564)
  line L134 (-43, 90.8564) -> (-44.5, 93.4545)
  line L135 (-44.5, 93.4545) -> (-47.5, 93.4545)
  line L136 (-47.5, 93.4545) -> (-49, 90.8564)
  line L137 (-49, 90.8564) -> (-47.5, 88.2583)
  line L138 (-79.5, 93.4545) -> (-81, 90.8564)
  line L139 (-81, 90.8564) -> (-79.5, 88.2583)
  line L140 (-79.5, 88.2583) -> (-76.5, 88.2583)
  line L141 (-76.5, 88.2583) -> (-75, 90.8564)
  line L142 (-75, 90.8564) -> (-76.5, 93.4545)
  line L143 (-76.5, 93.4545) -> (-79.5, 93.4545)
  line L144 (-59.5, 81.3301) -> (-56.5, 81.3301)
  line L145 (-56.5, 81.3301) -> (-55, 83.9282)
  line L146 (-55, 83.9282) -> (-56.5, 86.5263)
  line L147 (-56.5, 86.5263) -> (-59.5, 86.5263)
  line L148 (-59.5, 86.5263) -> (-61, 83.9282)
  line L149 (-61, 83.9282) -> (-59.5, 81.3301)
  line L150 (-71, 83.9282) -> (-72.5, 86.5263)
  line L151 (-72.5, 86.5263) -> (-75.5, 86.5263)
  line L152 (-75.5, 86.5263) -> (-77, 83.9282)
  line L153 (-77, 83.9282) -> (-75.5, 81.3301)
  line L154 (-75.5, 81.3301) -> (-72.5, 81.3301)
  line L155 (-72.5, 81.3301) -> (-71, 83.9282)
  line L156 (-7.5, 79.4545) -> (-9, 76.8564)
  line L157 (-9, 76.8564) -> (-7.5, 74.2583)
  line L158 (-7.5, 74.2583) -> (-4.5, 74.2583)
  line L159 (-4.5, 74.2583) -> (-3, 76.8564)
  line L160 (-3, 76.8564) -> (-4.5, 79.4545)
  line L161 (-4.5, 79.4545) -> (-7.5, 79.4545)
  line L162 (-31.5, 74.2583) -> (-28.5, 74.2583)
  line L163 (-28.5, 74.2583) -> (-27, 76.8564)
  line L164 (-27, 76.8564) -> (-28.5, 79.4545)
  line L165 (-28.5, 79.4545) -> (-31.5, 79.4545)
  line L166 (-31.5, 79.4545) -> (-33, 76.8564)
  line L167 (-33, 76.8564) -> (-31.5, 74.2583)
  line L168 (-19.5, 72.5263) -> (-21, 69.9282)
  line L169 (-21, 69.9282) -> (-19.5, 67.3301)
  line L170 (-19.5, 67.3301) -> (-16.5, 67.3301)
  line L171 (-16.5, 67.3301) -> (-15, 69.9282)
  line L172 (-15, 69.9282) -> (-16.5, 72.5263)
  line L173 (-16.5, 72.5263) -> (-19.5, 72.5263)
  line L174 (-27.5, 67.3301) -> (-24.5, 67.3301)
  line L175 (-24.5, 67.3301) -> (-23, 69.9282)
  line L176 (-23, 69.9282) -> (-24.5, 72.5263)
  line L177 (-24.5, 72.5263) -> (-27.5, 72.5263)
  line L178 (-27.5, 72.5263) -> (-29, 69.9282)
  line L179 (-29, 69.9282) -> (-27.5, 67.3301)
  line L180 (-39, 69.9282) -> (-40.5, 72.5263)
  line L181 (-40.5, 72.5263) -> (-43.5, 72.5263)
  line L182 (-43.5, 72.5263) -> (-45, 69.9282)
  line L183 (-45, 69.9282) -> (-43.5, 67.3301)
  line L184 (-43.5, 67.3301) -> (-40.5, 67.3301)
  line L185 (-40.5, 67.3301) -> (-39, 69.9282)
  line L186 (-63.5, 74.2583) -> (-60.5, 74.2583)
  line L187 (-60.5, 74.2583) -> (-59, 76.8564)
  line L188 (-59, 76.8564) -> (-60.5, 79.4545)
  line L189 (-60.5, 79.4545) -> (-63.5, 79.4545)
  line L190 (-63.5, 79.4545) -> (-65, 76.8564)
  line L191 (-65, 76.8564) -> (-63.5, 74.2583)
  line L192 (-47.5, 74.2583) -> (-44.5, 74.2583)
  line L193 (-44.5, 74.2583) -> (-43, 76.8564)
  line L194 (-43, 76.8564) -> (-44.5, 79.4545)
  line L195 (-44.5, 79.4545) -> (-47.5, 79.4545)
  line L196 (-47.5, 79.4545) -> (-49, 76.8564)
  line L197 (-49, 76.8564) -> (-47.5, 74.2583)
  line L198 (-79.5, 79.4545) -> (-81, 76.8564)
  line L199 (-81, 76.8564) -> (-79.5, 74.2583)
  line L200 (-79.5, 74.2583) -> (-76.5, 74.2583)
  line L201 (-76.5, 74.2583) -> (-75, 76.8564)
  line L202 (-75, 76.8564) -> (-76.5, 79.4545)
  line L203 (-76.5, 79.4545) -> (-79.5, 79.4545)
  line L204 (-59.5, 67.3301) -> (-56.5, 67.3301)
  line L205 (-56.5, 67.3301) -> (-55, 69.9282)
  line L206 (-55, 69.9282) -> (-56.5, 72.5263)
  line L207 (-56.5, 72.5263) -> (-59.5, 72.5263)
  line L208 (-59.5, 72.5263) -> (-61, 69.9282)
  line L209 (-61, 69.9282) -> (-59.5, 67.3301)
  line L210 (-71, 69.9282) -> (-72.5, 72.5263)
  line L211 (-72.5, 72.5263) -> (-75.5, 72.5263)
  line L212 (-75.5, 72.5263) -> (-77, 69.9282)
  line L213 (-77, 69.9282) -> (-75.5, 67.3301)
  line L214 (-75.5, 67.3301) -> (-72.5, 67.3301)
  line L215 (-72.5, 67.3301) -> (-71, 69.9282)
  line L216 (-7.5, 65.4545) -> (-9, 62.8564)
  line L217 (-9, 62.8564) -> (-7.5, 60.2583)
  line L218 (-7.5, 60.2583) -> (-4.5, 60.2583)
  line L219 (-4.5, 60.2583) -> (-3, 62.8564)
  line L220 (-3, 62.8564) -> (-4.5, 65.4545)
  line L221 (-4.5, 65.4545) -> (-7.5, 65.4545)
  line L222 (-31.5, 60.2583) -> (-28.5, 60.2583)
  line L223 (-28.5, 60.2583) -> (-27, 62.8564)
  line L224 (-27, 62.8564) -> (-28.5, 65.4545)
  line L225 (-28.5, 65.4545) -> (-31.5, 65.4545)
  line L226 (-31.5, 65.4545) -> (-33, 62.8564)
  line L227 (-33, 62.8564) -> (-31.5, 60.2583)
  line L228 (-19.5, 58.5263) -> (-21, 55.9282)
  line L229 (-21, 55.9282) -> (-19.5, 53.3301)
  line L230 (-19.5, 53.3301) -> (-16.5, 53.3301)
  line L231 (-16.5, 53.3301) -> (-15, 55.9282)
  line L232 (-15, 55.9282) -> (-16.5, 58.5263)
  line L233 (-16.5, 58.5263) -> (-19.5, 58.5263)
  line L234 (-27.5, 53.3301) -> (-24.5, 53.3301)
  line L235 (-24.5, 53.3301) -> (-23, 55.9282)
  line L236 (-23, 55.9282) -> (-24.5, 58.5263)
  line L237 (-24.5, 58.5263) -> (-27.5, 58.5263)
  line L238 (-27.5, 58.5263) -> (-29, 55.9282)
  line L239 (-29, 55.9282) -> (-27.5, 53.3301)
  line L240 (-39, 55.9282) -> (-40.5, 58.5263)
  line L241 (-40.5, 58.5263) -> (-43.5, 58.5263)
  line L242 (-43.5, 58.5263) -> (-45, 55.9282)
  line L243 (-45, 55.9282) -> (-43.5, 53.3301)
  line L244 (-43.5, 53.3301) -> (-40.5, 53.3301)
  line L245 (-40.5, 53.3301) -> (-39, 55.9282)
  line L246 (-63.5, 60.2583) -> (-60.5, 60.2583)
  line L247 (-60.5, 60.2583) -> (-59, 62.8564)
  line L248 (-59, 62.8564) -> (-60.5, 65.4545)
  line L249 (-60.5, 65.4545) -> (-63.5, 65.4545)
  line L250 (-63.5, 65.4545) -> (-65, 62.8564)
  line L251 (-65, 62.8564) -> (-63.5, 60.2583)
  line L252 (-47.5, 60.2583) -> (-44.5, 60.2583)
  line L253 (-44.5, 60.2583) -> (-43, 62.8564)
  line L254 (-43, 62.8564) -> (-44.5, 65.4545)
  line L255 (-44.5, 65.4545) -> (-47.5, 65.4545)
  line L256 (-47.5, 65.4545) -> (-49, 62.8564)
  line L257 (-49, 62.8564) -> (-47.5, 60.2583)
  line L258 (-79.5, 65.4545) -> (-81, 62.8564)
  line L259 (-81, 62.8564) -> (-79.5, 60.2583)
  line L260 (-79.5, 60.2583) -> (-76.5, 60.2583)
  line L261 (-76.5, 60.2583) -> (-75, 62.8564)
  line L262 (-75, 62.8564) -> (-76.5, 65.4545)
  line L263 (-76.5, 65.4545) -> (-79.5, 65.4545)
  line L264 (-59.5, 53.3301) -> (-56.5, 53.3301)
  line L265 (-56.5, 53.3301) -> (-55, 55.9282)
  line L266 (-55, 55.9282) -> (-56.5, 58.5263)
  line L267 (-56.5, 58.5263) -> (-59.5, 58.5263)
  line L268 (-59.5, 58.5263) -> (-61, 55.9282)
  line L269 (-61, 55.9282) -> (-59.5, 53.3301)
  line L270 (-71, 55.9282) -> (-72.5, 58.5263)
  line L271 (-72.5, 58.5263) -> (-75.5, 58.5263)
  line L272 (-75.5, 58.5263) -> (-77, 55.9282)
  line L273 (-77, 55.9282) -> (-75.5, 53.3301)
  line L274 (-75.5, 53.3301) -> (-72.5, 53.3301)
  line L275 (-72.5, 53.3301) -> (-71, 55.9282)
  line L276 (-7.5, 51.4545) -> (-9, 48.8564)
  line L277 (-9, 48.8564) -> (-7.5, 46.2583)
  line L278 (-7.5, 46.2583) -> (-4.5, 46.2583)
  line L279 (-4.5, 46.2583) -> (-3, 48.8564)
  line L280 (-3, 48.8564) -> (-4.5, 51.4545)
  line L281 (-4.5, 51.4545) -> (-7.5, 51.4545)
  line L282 (-31.5, 46.2583) -> (-28.5, 46.2583)
  line L283 (-28.5, 46.2583) -> (-27, 48.8564)
  line L284 (-27, 48.8564) -> (-28.5, 51.4545)
  line L285 (-28.5, 51.4545) -> (-31.5, 51.4545)
  line L286 (-31.5, 51.4545) -> (-33, 48.8564)
  line L287 (-33, 48.8564) -> (-31.5, 46.2583)
  line L288 (-19.5, 44.5263) -> (-21, 41.9282)
  line L289 (-21, 41.9282) -> (-19.5, 39.3301)
  line L290 (-19.5, 39.3301) -> (-16.5, 39.3301)
  line L291 (-16.5, 39.3301) -> (-15, 41.9282)
  line L292 (-15, 41.9282) -> (-16.5, 44.5263)
  line L293 (-16.5, 44.5263) -> (-19.5, 44.5263)
  line L294 (-27.5, 39.3301) -> (-24.5, 39.3301)
  line L295 (-24.5, 39.3301) -> (-23, 41.9282)
  line L296 (-23, 41.9282) -> (-24.5, 44.5263)
  line L297 (-24.5, 44.5263) -> (-27.5, 44.5263)
  line L298 (-27.5, 44.5263) -> (-29, 41.9282)
  line L299 (-29, 41.9282) -> (-27.5, 39.3301)
  line L300 (-39, 41.9282) -> (-40.5, 44.5263)
  line L301 (-40.5, 44.5263) -> (-43.5, 44.5263)
  line L302 (-43.5, 44.5263) -> (-45, 41.9282)
  line L303 (-45, 41.9282) -> (-43.5, 39.3301)
  line L304 (-43.5, 39.3301) -> (-40.5, 39.3301)
  line L305 (-40.5, 39.3301) -> (-39, 41.9282)
  line L306 (-63.5, 46.2583) -> (-60.5, 46.2583)
  line L307 (-60.5, 46.2583) -> (-59, 48.8564)
  line L308 (-59, 48.8564) -> (-60.5, 51.4545)
  line L309 (-60.5, 51.4545) -> (-63.5, 51.4545)
  line L310 (-63.5, 51.4545) -> (-65, 48.8564)
  line L311 (-65, 48.8564) -> (-63.5, 46.2583)
  line L312 (-47.5, 46.2583) -> (-44.5, 46.2583)
  line L313 (-44.5, 46.2583) -> (-43, 48.8564)
  line L314 (-43, 48.8564) -> (-44.5, 51.4545)
  line L315 (-44.5, 51.4545) -> (-47.5, 51.4545)
  line L316 (-47.5, 51.4545) -> (-49, 48.8564)
  line L317 (-49, 48.8564) -> (-47.5, 46.2583)
  line L318 (-79.5, 51.4545) -> (-81, 48.8564)
  line L319 (-81, 48.8564) -> (-79.5, 46.2583)
  line L320 (-79.5, 46.2583) -> (-76.5, 46.2583)
  line L321 (-76.5, 46.2583) -> (-75, 48.8564)
  line L322 (-75, 48.8564) -> (-76.5, 51.4545)
  line L323 (-76.5, 51.4545) -> (-79.5, 51.4545)
  line L324 (-59.5, 39.3301) -> (-56.5, 39.3301)
  line L325 (-56.5, 39.3301) -> (-55, 41.9282)
  line L326 (-55, 41.9282) -> (-56.5, 44.5263)
  line L327 (-56.5, 44.5263) -> (-59.5, 44.5263)
  line L328 (-59.5, 44.5263) -> (-61, 41.9282)
  line L329 (-61, 41.9282) -> (-59.5, 39.3301)
  line L330 (-71, 41.9282) -> (-72.5, 44.5263)
  line L331 (-72.5, 44.5263) -> (-75.5, 44.5263)
  line L332 (-75.5, 44.5263) -> (-77, 41.9282)
  line L333 (-77, 41.9282) -> (-75.5, 39.3301)
  line L334 (-75.5, 39.3301) -> (-72.5, 39.3301)
  line L335 (-72.5, 39.3301) -> (-71, 41.9282)
  line L336 (-7.5, 37.4545) -> (-9, 34.8564)
  line L337 (-9, 34.8564) -> (-7.5, 32.2583)
  line L338 (-7.5, 32.2583) -> (-4.5, 32.2583)
  line L339 (-4.5, 32.2583) -> (-3, 34.8564)
  line L340 (-3, 34.8564) -> (-4.5, 37.4545)
  line L341 (-4.5, 37.4545) -> (-7.5, 37.4545)
  line L342 (-31.5, 32.2583) -> (-28.5, 32.2583)
  line L343 (-28.5, 32.2583) -> (-27, 34.8564)
  line L344 (-27, 34.8564) -> (-28.5, 37.4545)
  line L345 (-28.5, 37.4545) -> (-31.5, 37.4545)
  line L346 (-31.5, 37.4545) -> (-33, 34.8564)
  line L347 (-33, 34.8564) -> (-31.5, 32.2583)
  line L348 (-19.5, 30.5263) -> (-21, 27.9282)
  line L349 (-21, 27.9282) -> (-19.5, 25.3301)
  line L350 (-19.5, 25.3301) -> (-16.5, 25.3301)
  line L351 (-16.5, 25.3301) -> (-15, 27.9282)
  line L352 (-15, 27.9282) -> (-16.5, 30.5263)
  line L353 (-16.5, 30.5263) -> (-19.5, 30.5263)
  line L354 (-27.5, 25.3301) -> (-24.5, 25.3301)
  line L355 (-24.5, 25.3301) -> (-23, 27.9282)
  line L356 (-23, 27.9282) -> (-24.5, 30.5263)
  line L357 (-24.5, 30.5263) -> (-27.5, 30.5263)
  line L358 (-27.5, 30.5263) -> (-29, 27.9282)
  line L359 (-29, 27.9282) -> (-27.5, 25.3301)
  line L360 (-39, 27.9282) -> (-40.5, 30.5263)
  line L361 (-40.5, 30.5263) -> (-43.5, 30.5263)
  line L362 (-43.5, 30.5263) -> (-45, 27.9282)
  line L363 (-45, 27.9282) -> (-43.5, 25.3301)
  line L364 (-43.5, 25.3301) -> (-40.5, 25.3301)
  line L365 (-40.5, 25.3301) -> (-39, 27.9282)
  line L366 (-63.5, 32.2583) -> (-60.5, 32.2583)
  line L367 (-60.5, 32.2583) -> (-59, 34.8564)
  line L368 (-59, 34.8564) -> (-60.5, 37.4545)
  line L369 (-60.5, 37.4545) -> (-63.5, 37.4545)
  line L370 (-63.5, 37.4545) -> (-65, 34.8564)
  line L371 (-65, 34.8564) -> (-63.5, 32.2583)
  line L372 (-47.5, 32.2583) -> (-44.5, 32.2583)
  line L373 (-44.5, 32.2583) -> (-43, 34.8564)
  line L374 (-43, 34.8564) -> (-44.5, 37.4545)
  line L375 (-44.5, 37.4545) -> (-47.5, 37.4545)
  line L376 (-47.5, 37.4545) -> (-49, 34.8564)
  line L377 (-49, 34.8564) -> (-47.5, 32.2583)
  line L378 (-79.5, 37.4545) -> (-81, 34.8564)
  line L379 (-81, 34.8564) -> (-79.5, 32.2583)
  line L380 (-79.5, 32.2583) -> (-76.5, 32.2583)
  line L381 (-76.5, 32.2583) -> (-75, 34.8564)
  line L382 (-75, 34.8564) -> (-76.5, 37.4545)
  line L383 (-76.5, 37.4545) -> (-79.5, 37.4545)
  line L384 (-59.5, 25.3301) -> (-56.5, 25.3301)
  line L385 (-56.5, 25.3301) -> (-55, 27.9282)
  line L386 (-55, 27.9282) -> (-56.5, 30.5263)
  line L387 (-56.5, 30.5263) -> (-59.5, 30.5263)
  line L388 (-59.5, 30.5263) -> (-61, 27.9282)
  line L389 (-61, 27.9282) -> (-59.5, 25.3301)
  line L390 (-71, 27.9282) -> (-72.5, 30.5263)
  line L391 (-72.5, 30.5263) -> (-75.5, 30.5263)
  line L392 (-75.5, 30.5263) -> (-77, 27.9282)
  line L393 (-77, 27.9282) -> (-75.5, 25.3301)
  line L394 (-75.5, 25.3301) -> (-72.5, 25.3301)
  line L395 (-72.5, 25.3301) -> (-71, 27.9282)
  line L396 (-3, 20.8564) -> (-4.5, 23.4545)
  line L397 (-4.5, 23.4545) -> (-7.5, 23.4545)
  line L398 (-7.5, 23.4545) -> (-9, 20.8564)
  line L399 (-9, 20.8564) -> (-7.5, 18.2583)
  line L400 (-7.5, 18.2583) -> (-4.5, 18.2583)
  line L401 (-4.5, 18.2583) -> (-3, 20.8564)
  line L402 (-67, 20.8564) -> (-68.5, 23.4545)
  line L403 (-68.5, 23.4545) -> (-71.5, 23.4545)
  line L404 (-71.5, 23.4545) -> (-73, 20.8564)
  line L405 (-73, 20.8564) -> (-71.5, 18.2583)
  line L406 (-71.5, 18.2583) -> (-68.5, 18.2583)
  line L407 (-68.5, 18.2583) -> (-67, 20.8564)
  line L408 (-51, 20.8564) -> (-52.5, 23.4545)
  line L409 (-52.5, 23.4545) -> (-55.5, 23.4545)
  line L410 (-55.5, 23.4545) -> (-57, 20.8564)
  line L411 (-57, 20.8564) -> (-55.5, 18.2583)
  line L412 (-55.5, 18.2583) -> (-52.5, 18.2583)
  line L413 (-52.5, 18.2583) -> (-51, 20.8564)
  line L414 (-35, 20.8564) -> (-36.5, 23.4545)
  line L415 (-36.5, 23.4545) -> (-39.5, 23.4545)
  line L416 (-39.5, 23.4545) -> (-41, 20.8564)
  line L417 (-41, 20.8564) -> (-39.5, 18.2583)
  line L418 (-39.5, 18.2583) -> (-36.5, 18.2583)
  line L419 (-36.5, 18.2583) -> (-35, 20.8564)
  line L420 (-19, 20.8564) -> (-20.5, 23.4545)
  line L421 (-20.5, 23.4545) -> (-23.5, 23.4545)
  line L422 (-23.5, 23.4545) -> (-25, 20.8564)
  line L423 (-25, 20.8564) -> (-23.5, 18.2583)
  line L424 (-23.5, 18.2583) -> (-20.5, 18.2583)
  line L425 (-20.5, 18.2583) -> (-19, 20.8564)
  line L426 (-85, 13.9282) -> (-83.5, 11.3301)
  line L427 (-83.5, 11.3301) -> (-80.5, 11.3301)
  line L428 (-80.5, 11.3301) -> (-79, 13.9282)
  line L429 (-79, 13.9282) -> (-80.5, 16.5263)
  line L430 (-80.5, 16.5263) -> (-83.5, 16.5263)
  line L431 (-83.5, 16.5263) -> (-85, 13.9282)
  line L432 (-63, 13.9282) -> (-64.5, 16.5263)
  line L433 (-64.5, 16.5263) -> (-67.5, 16.5263)
  line L434 (-67.5, 16.5263) -> (-69, 13.9282)
  line L435 (-69, 13.9282) -> (-67.5, 11.3301)
  line L436 (-67.5, 11.3301) -> (-64.5, 11.3301)
  line L437 (-64.5, 11.3301) -> (-63, 13.9282)
  line L438 (-47, 13.9282) -> (-48.5, 16.5263)
  line L439 (-48.5, 16.5263) -> (-51.5, 16.5263)
  line L440 (-51.5, 16.5263) -> (-53, 13.9282)
  line L441 (-53, 13.9282) -> (-51.5, 11.3301)
  line L442 (-51.5, 11.3301) -> (-48.5, 11.3301)
  line L443 (-48.5, 11.3301) -> (-47, 13.9282)
  line L444 (-31, 13.9282) -> (-32.5, 16.5263)
  line L445 (-32.5, 16.5263) -> (-35.5, 16.5263)
  line L446 (-35.5, 16.5263) -> (-37, 13.9282)
  line L447 (-37, 13.9282) -> (-35.5, 11.3301)
  line L448 (-35.5, 11.3301) -> (-32.5, 11.3301)
  line L449 (-32.5, 11.3301) -> (-31, 13.9282)
  line L450 (-15, 13.9282) -> (-16.5, 16.5263)
  line L451 (-16.5, 16.5263) -> (-19.5, 16.5263)
  line L452 (-19.5, 16.5263) -> (-21, 13.9282)
  line L453 (-21, 13.9282) -> (-19.5, 11.3301)
  line L454 (-19.5, 11.3301) -> (-16.5, 11.3301)
  line L455 (-16.5, 11.3301) -> (-15, 13.9282)
  line L456 (-59, 7) -> (-60.5, 9.5981)
  line L457 (-60.5, 9.5981) -> (-63.5, 9.5981)
  line L458 (-63.5, 9.5981) -> (-65, 7)
  line L459 (-65, 7) -> (-63.5, 4.4019)
  line L460 (-63.5, 4.4019) -> (-60.5, 4.4019)
  line L461 (-60.5, 4.4019) -> (-59, 7)
  line L462 (-43, 7) -> (-44.5, 9.5981)
  line L463 (-44.5, 9.5981) -> (-47.5, 9.5981)
  line L464 (-47.5, 9.5981) -> (-49, 7)
  line L465 (-49, 7) -> (-47.5, 4.4019)
  line L466 (-47.5, 4.4019) -> (-44.5, 4.4019)
  line L467 (-44.5, 4.4019) -> (-43, 7)
  line L468 (-27, 7) -> (-28.5, 9.5981)
  line L469 (-28.5, 9.5981) -> (-31.5, 9.5981)
  line L470 (-31.5, 9.5981) -> (-33, 7)
  line L471 (-33, 7) -> (-31.5, 4.4019)
  line L472 (-31.5, 4.4019) -> (-28.5, 4.4019)
  line L473 (-28.5, 4.4019) -> (-27, 7)
  line L474 (-19, 7) -> (-20.5, 9.5981)
  line L475 (-20.5, 9.5981) -> (-23.5, 9.5981)
  line L476 (-23.5, 9.5981) -> (-25, 7)
  line L477 (-25, 7) -> (-23.5, 4.4019)
  line L478 (-23.5, 4.4019) -> (-20.5, 4.4019)
  line L479 (-20.5, 4.4019) -> (-19, 7)
  line L480 (-35, 7) -> (-36.5, 9.5981)
  line L481 (-36.5, 9.5981) -> (-39.5, 9.5981)
  line L482 (-39.5, 9.5981) -> (-41, 7)
  line L483 (-41, 7) -> (-39.5, 4.4019)
  line L484 (-39.5, 4.4019) -> (-36.5, 4.4019)
  line L485 (-36.5, 4.4019) -> (-35, 7)
  line L486 (-51, 7) -> (-52.5, 9.5981)
  line L487 (-52.5, 9.5981) -> (-55.5, 9.5981)
  line L488 (-55.5, 9.5981) -> (-57, 7)
  line L489 (-57, 7) -> (-55.5, 4.4019)
  line L490 (-55.5, 4.4019) -> (-52.5, 4.4019)
  line L491 (-52.5, 4.4019) -> (-51, 7)
  line L492 (-67, 7) -> (-68.5, 9.5981)
  line L493 (-68.5, 9.5981) -> (-71.5, 9.5981)
  line L494 (-71.5, 9.5981) -> (-73, 7)
  line L495 (-73, 7) -> (-71.5, 4.4019)
  line L496 (-71.5, 4.4019) -> (-68.5, 4.4019)
  line L497 (-68.5, 4.4019) -> (-67, 7)
  line L498 (-7, 13.9282) -> (-8.5, 16.5263)
  line L499 (-8.5, 16.5263) -> (-11.5, 16.5263)
  line L500 (-11.5, 16.5263) -> (-13, 13.9282)
  line L501 (-13, 13.9282) -> (-11.5, 11.3301)
  line L502 (-11.5, 11.3301) -> (-8.5, 11.3301)
  line L503 (-8.5, 11.3301) -> (-7, 13.9282)
  line L504 (-23, 13.9282) -> (-24.5, 16.5263)
  line L505 (-24.5, 16.5263) -> (-27.5, 16.5263)
  line L506 (-27.5, 16.5263) -> (-29, 13.9282)
  line L507 (-29, 13.9282) -> (-27.5, 11.3301)
  line L508 (-27.5, 11.3301) -> (-24.5, 11.3301)
  line L509 (-24.5, 11.3301) -> (-23, 13.9282)
  line L510 (-39, 13.9282) -> (-40.5, 16.5263)
  line L511 (-40.5, 16.5263) -> (-43.5, 16.5263)
  line L512 (-43.5, 16.5263) -> (-45, 13.9282)
  line L513 (-45, 13.9282) -> (-43.5, 11.3301)
  line L514 (-43.5, 11.3301) -> (-40.5, 11.3301)
  line L515 (-40.5, 11.3301) -> (-39, 13.9282)
  line L516 (-55, 13.9282) -> (-56.5, 16.5263)
  line L517 (-56.5, 16.5263) -> (-59.5, 16.5263)
  line L518 (-59.5, 16.5263) -> (-61, 13.9282)
  line L519 (-61, 13.9282) -> (-59.5, 11.3301)
  line L520 (-59.5, 11.3301) -> (-56.5, 11.3301)
  line L521 (-56.5, 11.3301) -> (-55, 13.9282)
  line L522 (-71, 13.9282) -> (-72.5, 16.5263)
  line L523 (-72.5, 16.5263) -> (-75.5, 16.5263)
  line L524 (-75.5, 16.5263) -> (-77, 13.9282)
  line L525 (-77, 13.9282) -> (-75.5, 11.3301)
  line L526 (-75.5, 11.3301) -> (-72.5, 11.3301)
  line L527 (-72.5, 11.3301) -> (-71, 13.9282)
  line L528 (-11, 20.8564) -> (-12.5, 23.4545)
  line L529 (-12.5, 23.4545) -> (-15.5, 23.4545)
  line L530 (-15.5, 23.4545) -> (-17, 20.8564)
  line L531 (-17, 20.8564) -> (-15.5, 18.2583)
  line L532 (-15.5, 18.2583) -> (-12.5, 18.2583)
  line L533 (-12.5, 18.2583) -> (-11, 20.8564)
  line L534 (-27, 20.8564) -> (-28.5, 23.4545)
  line L535 (-28.5, 23.4545) -> (-31.5, 23.4545)
  line L536 (-31.5, 23.4545) -> (-33, 20.8564)
  line L537 (-33, 20.8564) -> (-31.5, 18.2583)
  line L538 (-31.5, 18.2583) -> (-28.5, 18.2583)
  line L539 (-28.5, 18.2583) -> (-27, 20.8564)
  line L540 (-43, 20.8564) -> (-44.5, 23.4545)
  line L541 (-44.5, 23.4545) -> (-47.5, 23.4545)
  line L542 (-47.5, 23.4545) -> (-49, 20.8564)
  line L543 (-49, 20.8564) -> (-47.5, 18.2583)
  line L544 (-47.5, 18.2583) -> (-44.5, 18.2583)